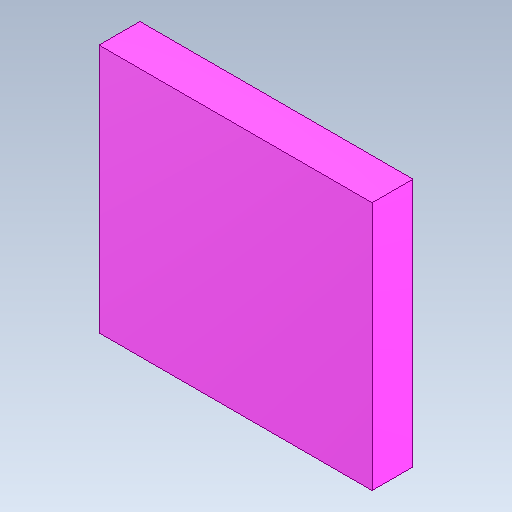
# Autodesk Inventor part: SW-PF0_B3F-10XX
Saved by Autodesk Inventor 2021 (Build 250183000, 183)
## iProperties
Created: 2020-11-03
Part Number: SW-PF0_B3F-10XX
Material: Generic
Document SubType Name: Modeling
Designer: faiya
Density: 1 g/cm^3
Appearance: B3F-10XX, SW-PF0_B3F-10XX
Author: faiya
Autodesk Inventor part; units mm, degrees
ref_plane "YZ Plane" through (0, 0, 0) normal (1, 0, 0) x (0, 1, 0)
ref_plane "XZ Plane" through (0, 0, 0) normal (0, 1, 0) x (-1, 0, 0)
ref_plane "XY Plane" through (0, 0, 0) normal (0, 0, 1) x (1, 0, 0)
sketch "B3F-10XX, SW-PF0_B3F-10XX_64" plane through (0, 0, 0) normal (0, 0, 1) x (1, 0, 0)
  line L0 (-3.302, 3.048) -> (3.3782, 3.048)
  line L1 (3.3782, 3.048) -> (3.3782, -3.048)
  line L2 (3.3782, -3.048) -> (-3.302, -3.048)
  line L3 (-3.302, -3.048) -> (-3.302, 3.048)
  constraints: 8 end point
extrude "Extrusion1" add sketch "B3F-10XX, SW-PF0_B3F-10XX_64" along normal blind 1
body "Solid1"
